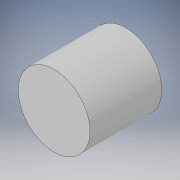
# Autodesk Inventor part: test
Saved by Autodesk Inventor 2019.3 (Build 233278000, 278)
## iProperties
Created: 2019-08-29
Part Number: test
Material: Generic
Document SubType Name: Modeling
Designer: Frienddo
Density: 1 g/cm^3
Appearance: Default
Author: Frienddo
Autodesk Inventor part; units mm, degrees
ref_plane "YZ Plane" through (0, 0, 0) normal (1, 0, 0) x (0, 1, 0)
ref_plane "XZ Plane" through (0, 0, 0) normal (0, 1, 0) x (-1, 0, 0)
ref_plane "XY Plane" through (0, 0, 0) normal (0, 0, 1) x (1, 0, 0)
sketch "Sketch2" plane through (0, 0, 0) normal (0, 0, 1) x (1, 0, 0)
  circle A0 centre (0, 0) radius 333
  dimension "d0" = 666
  constraints: 1 centre point, 1 coincident
  measures "d0" diameter of A0
extrude "Extrusion1" add sketch "Sketch2" along normal mid plane 666
equation "\"d0\" = diam"
equation "\"d1\" = thickness"
equation "\"diam\" = 666"
equation "\"thickness\" = 666"
body "Solid1"
